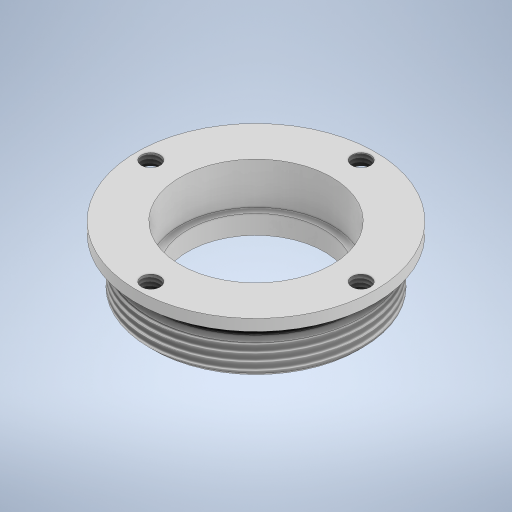
# Autodesk Inventor part: 018
Saved by Autodesk Inventor 2023 (Build 270158000, 158)
## iProperties
Created: 2021-11-15
Part Number: 018
Material: Generic
Document SubType Name: Modeling
Designer: vinicius.miguel
Density: 1 g/cm^3
Appearance: Default
Mass: 2.32398 g
Surface Area: 31.3827 cm^2
Volume: 2.32398 cm^3
Author: vinicius.miguel
Autodesk Inventor part; units mm, degrees
ref_plane "YZ Plane" through (0, 0, 0) normal (1, 0, 0) x (0, 1, 0)
ref_plane "XZ Plane" through (0, 0, 0) normal (0, 1, 0) x (-1, 0, 0)
ref_plane "XY Plane" through (0, 0, 0) normal (0, 0, 1) x (1, 0, 0)
sketch "Sketch1" plane through (0, 0, 0) normal (0, 0, 1) x (1, 0, 0)
  line L0 (0, 0) -> (0, 8)
  line L1 (9, 0) -> (9, 2.5)
  line L2 (9, 2.5) -> (10, 2.5)
  line L3 (10, 2.5) -> (10, 8)
  line L4 (10, 8) -> (12, 8)
  line L5 (12, 8) -> (12, 4.5)
  line L6 (12, 4.5) -> (14, 4.5)
  line L7 (14, 4.5) -> (14, 0)
  line L8 (14, 0) -> (9, 0)
  line L9 (12, 8) -> (15.75, 8)
  line L10 (15.75, 8) -> (15.75, 6.5)
  line L11 (15.75, 6.5) -> (12, 6.5)
  dimension "d0" = 18
  dimension "d2" = 2
  dimension "d3" = 2
  dimension "d4" = 4.5
  dimension "d5" = 20
  dimension "d13" = 28
  dimension "d14" = 1.5
  dimension "d15" = 31.5
  dimension "d28" = 2
  constraints: 24 end point, 9 perpendicular, 2 horizontal alignment, 2 vertical, 1 horizontal, 1 point on line
  measures "d0" diameter of L1 L0
  measures "d2" distance between parallel lines of L5 L3
  measures "d3" distance between parallel lines of L6 L2
  measures "d4" distance between parallel lines of L6 L8
  measures "d5" diameter of L3 L0
  measures "d13" diameter of L7 L0
  measures "d14" distance of L9.end L10.end
  measures "d15" diameter of L10 L0
  measures "d28" distance between parallel lines of L6 L11
revolve "Revolution1" add sketch "Sketch1" angle 360 about axis through (0, 0, 0) along (0, 1, 0)
chamfer "Chamfer1" distance 0.5 angle 45 2 edges at (-14, 4.5, 0) (-14, 0, 0)
thread "Thread1" size "M28x1" class "6g" standard "ANSI Metric M Profile" full length
sketch "Sketch3" plane through (0, 8, 0) normal (0, 1, 0) x (1, 0, 0)
  circle A0 centre (0, 0) radius 15.75 projected
  circle A1 centre (0, 0) radius 12 projected
  line L0 (12, 0) -> (15.75, 0)
  point P0 (13.875, 0)
  constraints: 3 horizontal alignment, 2 end point, 1 horizontal, 1 midpoint, 2 other
hole "Hole2" at (13.875, 8, 0) direction (0, -1, 0) diameter 2.459 depth 1.5 thread size "M3x0.5" class "6H" standard "ISO Metric profile"
pattern_circular "Circular Pattern2" count 4 over 360 about axis through (0, 5.25, 0) along (0, -1, 0) of "Hole2"
equation "\"d3\" = d2"
body "Solid1"
